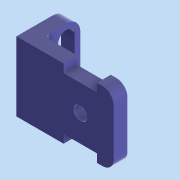
# Autodesk Inventor part: ejercicio 266
Saved by Autodesk Inventor 2018 (Build 220112000, 112)
## iProperties
Created: 2021-04-06
Part Number: ejercicio 266
Material: Thermoplastic Resin
Document SubType Name: Modeling
Designer: asus
Density: 1.28 g/cm^3
Appearance: Smooth - Black
Author: asus
Autodesk Inventor part; units mm, degrees
ref_plane "YZ Plane" through (0, 0, 0) normal (1, 0, 0) x (0, 1, 0)
ref_plane "XZ Plane" through (0, 0, 0) normal (0, 1, 0) x (-1, 0, 0)
ref_plane "XY Plane" through (0, 0, 0) normal (0, 0, 1) x (1, 0, 0)
sketch "Sketch1" plane through (0, 0, 0) normal (0, 1, 0) x (-1, 0, 0)
  line L0 (-17.5, -12.5) -> (17.5, -12.5)
  line L1 (17.5, -12.5) -> (17.5, 12.5)
  line L2 (17.5, 12.5) -> (-17.5, 12.5)
  line L3 (-17.5, 12.5) -> (-17.5, -12.5)
  line L4 (-17.5, -12.5) -> (17.5, 12.5) construction
  line L5 (17.5, -12.5) -> (-17.5, 12.5) construction
  line L6 (-17.5, 0) -> (17.5, 0) construction
  line L7 (0.5, 12.5) -> (0.5, 9.5)
  line L8 (0.5, 9.5) -> (-11.5, 9.5)
  line L9 (-11.5, 9.5) -> (-11.5, 12.5)
  line L10 (-11.5, 15.5) -> (0.5, 9.5) construction
  line L11 (0.5, 15.5) -> (-11.5, 9.5) construction
  line L12 (0.5, -12.5) -> (0.5, -9.5)
  line L13 (0.5, -9.5) -> (-11.5, -9.5)
  line L14 (-11.5, -9.5) -> (-11.5, -12.5)
  circle A0 centre (-5.5, 0) radius 4
  point P0 (0, 0)
  point P1 (-5.5, 12.5)
  dimension "d0" = 35
  dimension "d1" = 25
  dimension "d2" = 6
  dimension "d3" = 12
  dimension "d4" = 6
  dimension "d5" = 19
  dimension "d6" = 8
  constraints: 30 end point, 6 midpoint, 6 point on line, 3 parallel, 2 symmetric about line, 1 centre point, 1 horizontal, 1 perpendicular
  measures "d0" distance of L0.start L0.end
  measures "d1" distance of L0.end L1.end
  measures "d2" distance between parallel lines of L3 L9
  measures "d3" distance between parallel lines of L7 L9
  measures "d4" distance of L11.start L7.end
  measures "d5" distance between parallel lines of L13 L8
  measures "d6" diameter of A0
extrude "Extrusion1" add sketch "Sketch1" along normal blind 5 contours L3 L2 L9 L8 L7 L1 L0 L12 L13 L14
sketch "Sketch2" plane through (-17.5, 0, -12.5) normal (-1, 0, 0) x (0, 0, 1)
  line L0 (22, 0) -> (25, 0) projected
  line L1 (0, 0) -> (25, 0)
  line L2 (25, 0) -> (25, 18)
  line L3 (25, 18) -> (0, 18)
  line L4 (0, 18) -> (0, 0)
  point P0 (12.5, 0)
  dimension "d9" = 18
  dimension "d10" = 25
  constraints: 8 end point, 2 parallel, 1 horizontal, 1 perpendicular
  measures "d9" distance between parallel lines of L1 L3
  measures "d10" distance between parallel lines of L4 L2
extrude "Extrusion2" add sketch "Sketch2" against normal blind 5
sketch "Sketch3" plane through (-17.5, 0, -12.5) normal (-1, 0, 0) x (0, 0, 1)
  line L0 (5, 13) -> (20, 13) construction
  line L1 (5, 10) -> (20, 10)
  line L2 (20, 16) -> (5, 16)
  arc A0 (5, 16) -> (5, 10) centre (5, 13) ccw
  arc A1 (20, 10) -> (20, 16) centre (20, 13) ccw
  line L3 (0, 0) -> (0, 18) projected
  line L4 (25, 18) -> (0, 18) projected
  point P0 (12.5, 0)
  point P1 (12.5, 13)
  dimension "d16" = 12.5
  dimension "d17" = 15
  dimension "d18" = 5
  dimension "d19" = 3
  constraints: 8 end point, 4 point on circle, 4 tangent, 2 centre point, 1 horizontal, 1 midpoint, 1 parallel
  measures "d16" distance from line of L3 point (12.5, 13)
  measures "d17" distance of L0.start L0.end
  measures "d18" distance between parallel lines of L0 L4
  measures "d19" radius of A1
extrude "Extrusion3" cut sketch "Sketch3" against normal blind 5
sketch "Sketch4" plane through (0, 0, 0) normal (0, 1, 0) x (-1, 0, 0)
  circle A0 centre (-5.5, 0) radius 4 projected
  circle A1 centre (-5.5, 0) radius 2.5
  point P0 (0, 0)
  dimension "d22" = 5
  constraints: 1 centre point, 1 coincident
  measures "d22" diameter of A1
extrude "Extrusion4" add sketch "Sketch4" along normal blind 3
fillet "Fillet1" radius 5 2 edges at (-15, 18, 12.5) (-15, 18, -12.5)
fillet "Fillet2" radius 2 1 edges at (-12.5, 5, 0)
fillet "Fillet3" radius 4 2 edges at (17.5, 2.5, 12.5) (17.5, 2.5, -12.5)
body "Solid1"
